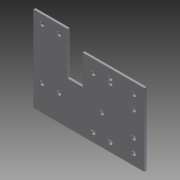
# Autodesk Inventor part: AS5-8-5-002
Saved by Autodesk Inventor 2011 SP1 (Build 150282100, 282)
## iProperties
Created: 2011-01-12
Part Number: AS5-8-5-002
Document SubType Name: Modeling
Designer: Christopher
Density: 1 g/cm^3
Author: Christopher
Autodesk Inventor part; units mm, degrees
ref_plane "YZ Plane" through (0, 0, 0) normal (1, 0, 0) x (0, 1, 0)
ref_plane "XZ Plane" through (0, 0, 0) normal (0, 1, 0) x (-1, 0, 0)
ref_plane "XY Plane" through (0, 0, 0) normal (0, 0, 1) x (1, 0, 0)
sketch "Sketch1" plane through (0, 0, 0) normal (0, 0, 1) x (1, 0, 0)
  line L0 (-59.7338, 79.3295) -> (-59.7338, -47.6705)
  line L1 (-59.7338, -47.6705) -> (67.2662, -47.6705)
  line L2 (67.2662, -47.6705) -> (67.2662, 60.2795)
  line L3 (67.2662, 60.2795) -> (13.2912, 60.2795)
  line L4 (13.2912, 60.2795) -> (13.2912, 15.8295)
  line L5 (13.2912, 15.8295) -> (-8.9338, 15.8295)
  line L6 (-8.9338, 15.8295) -> (-8.9338, 79.3295)
  line L7 (-8.9338, 79.3295) -> (-59.7338, 79.3295)
  line L8 (67.2662, 60.2795) -> (105.3662, 60.2795)
  line L9 (105.3662, 60.2795) -> (105.3662, -47.6705)
  line L10 (105.3662, -47.6705) -> (67.2662, -47.6705)
  point P0 (0, 0)
  point P1 (-47.0338, 66.6295)
  point P2 (54.5662, 47.5795)
  point P3 (41.8662, -3.2205)
  point P4 (54.5662, -34.9705)
  point P5 (-47.0338, -9.5705)
  point P6 (89.4658, -31.7955)
  point P7 (89.4658, -11.8057)
  point P8 (-21.6338, 66.6295)
  point P9 (-21.6338, -9.5705)
  point P10 (29.1662, 47.5795)
  point P11 (54.5662, -34.9705)
  point P12 (54.5662, -9.5705)
  point P13 (29.1662, -34.9705)
  point P14 (89.4658, 44.4045)
  point P15 (89.4658, 24.4147)
  dimension "d0" = 127
  dimension "d1" = 127
  dimension "d2" = 50.8
  dimension "d3" = 53.975
  dimension "d4" = 107.95
  dimension "d5" = 63.5
  dimension "d6" = 12.7
  dimension "d7" = 12.7
  dimension "d8" = 12.7
  dimension "d9" = 12.7
  dimension "d10" = 44.45
  dimension "d11" = 25.4
  dimension "d21" = 12.7
  dimension "d22" = 12.7
  dimension "d23" = 12.7
  dimension "d24" = 38.1
  dimension "d25" = 38.1
  dimension "d26" = 107.95
  dimension "d27" = 15.875
  dimension "d28" = 19.9898
  dimension "d38" = 15.9004
  dimension "d39" = 15.9004
  dimension "d40" = 12.7
  dimension "d41" = 12.7
  dimension "d42" = 25.4
  dimension "d43" = 76.2
  dimension "d44" = 12.7
  dimension "d46" = 12.7
  dimension "d47" = 25.4
  dimension "d48" = 38.1
  dimension "d49" = 12.7
  dimension "d50" = 12.7
  dimension "d51" = 38.1
  dimension "d52" = 25.4
  dimension "d54" = 15.875
  dimension "d55" = 19.9898
  dimension "d56" = 15.9004
  dimension "d57" = 15.9004
  constraints: 22 end point, 7 parallel, 2 perpendicular, 1 collinear, 1 point on line, 1 vertical
  measures "d0" distance of L0.start L0.end
  measures "d1" distance of L0.end L1.end
  measures "d2" distance of L6.end L0.start
  measures "d3" distance of L2.end L3.end
  measures "d4" distance of L1.end L2.end
  measures "d5" distance between parallel lines of L7 L5
  measures "d6" distance from line of L7 point (-47.034, 66.63)
  measures "d7" distance from line of L0 point (-47.034, 66.63)
  measures "d8" distance from line of L2 point (54.566, 47.58)
  measures "d9" distance from line of L3 point (54.566, 47.58)
  measures "d10" distance from line of L1 point (41.866, -3.22)
  measures "d11" distance from line of L2 point (41.866, -3.22)
  measures "d21" distance from line of L2 point (54.566, -34.97)
  measures "d22" distance from line of L1 point (54.566, -34.97)
  measures "d23" distance from line of L0 point (-47.034, -9.57)
  measures "d24" distance from line of L1 point (-47.034, -9.57)
  measures "d25" distance between parallel lines of L2 L9
  measures "d26" distance of L8.end L9.end
  measures "d27" distance from line of L10 point (89.466, -31.795)
  measures "d28" distance of point (89.466, -11.806) point (89.466, -31.795)
  measures "d38" distance from line of L9 point (89.466, -11.806)
  measures "d39" distance from line of L9 point (89.466, -31.795)
  measures "d40" distance from line of L6 point (-21.634, 66.63)
  measures "d41" distance from line of L7 point (-21.634, 66.63)
  measures "d42" distance of point (-21.634, -9.57) point (-47.034, -9.57)
  measures "d43" distance of point (-21.634, 66.63) point (-21.634, -9.57)
  measures "d44" distance from line of L3 point (29.166, 47.58)
  measures "d46" distance from line of L2 point (54.566, -9.57)
  measures "d47" distance of point (54.566, -34.97) point (54.566, -9.57)
  measures "d48" distance from line of L1 point (54.566, -9.57)
  measures "d49" distance from line of L1 point (54.566, -34.97)
  measures "d50" distance from line of L1 point (29.166, -34.97)
  measures "d51" distance from line of L2 point (29.166, -34.97)
  measures "d52" distance of point (54.566, 47.58) point (29.166, 47.58)
  measures "d54" distance from line of L8 point (89.466, 44.405)
  measures "d55" distance of point (89.466, 44.405) point (89.466, 24.415)
  measures "d56" distance from line of L9 point (89.466, 44.405)
  measures "d57" distance from line of L9 point (89.466, 24.415)
extrude "Extrusion1" add sketch "Sketch1" against normal blind 3.175 contours L7 L6 L5 L4 L3 L2 L1 L0
hole "Hole1" at (-47.0338, 66.6295, 0) at (54.5662, 47.5795, 0) at (41.8662, -3.2205, 0) at (-47.0338, -9.5705, 0) at (54.5662, -34.9705, 0) at (89.4658, -31.7955, 0) at (89.4658, -11.8057, 0) at (-21.6338, 66.6295, 0) at (-21.6338, -9.5705, 0) at (29.1662, 47.5795, 0) at (29.1662, -34.9705, 0) direction (0, 0, -1) diameter 6.35 depth 25.4 tip angle 118
extrude "Extrusion2" add sketch "Sketch1" against normal blind 3.175 contours L2 L8 L9 L10
hole "Hole2" at (89.4658, -11.8057, 0) at (89.4658, -31.7955, 0) at (89.4658, 24.4147, 0) at (89.4658, 44.4045, 0) direction (0, 0, -1) diameter 6.35 depth 25.4 tip angle 118
body "Solid1"
